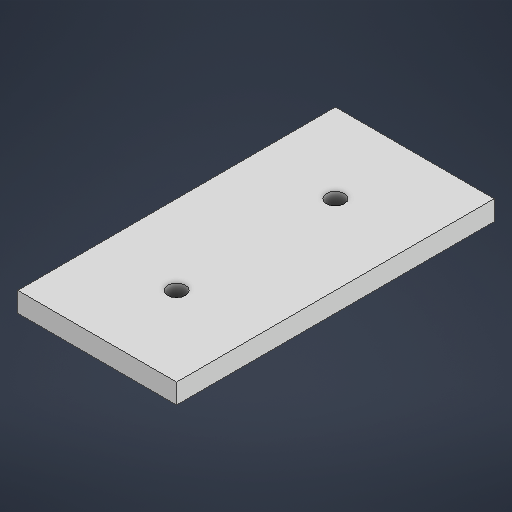
# Autodesk Inventor part: Bolt Slot Covers
Saved by Autodesk Inventor 2026.2 (Build 302298000, 298)
## iProperties
Created: 2026-05-27
Part Number: Bolt Slot Covers
Material: Generic
Document SubType Name: Modeling
Designer: mayhe
Density: 1 g/cm^3
Appearance: Default
Author: mayhe
Autodesk Inventor part; units mm, degrees
ref_plane "YZ Plane" through (0, 0, 0) normal (1, 0, 0) x (0, 1, 0)
ref_plane "XZ Plane" through (0, 0, 0) normal (0, 1, 0) x (-1, 0, 0)
ref_plane "XY Plane" through (0, 0, 0) normal (0, 0, 1) x (1, 0, 0)
sketch "Sketch1" plane through (0, 0, 0) normal (0, 1, 0) x (-1, 0, 0)
  line L0 (20, 40) -> (-20, 40)
  line L1 (-20, 40) -> (-20, -40)
  line L2 (-20, -40) -> (20, -40)
  line L3 (20, -40) -> (20, 40)
  line L4 (20, 40) -> (-20, -40) construction
  line L5 (-20, 40) -> (20, -40) construction
  circle A0 centre (0, 20) radius 2.25
  line L6 (20, 0) -> (36.628, 0)
  circle A1 centre (0, -20) radius 2.25
  point P0 (0, 0)
  dimension "d0" = 40
  dimension "d1" = 80
  dimension "d2" = 4.5
  dimension "d3" = 20
  constraints: 14 end point, 3 midpoint, 2 centre point, 2 horizontal, 2 parallel, 1 perpendicular, 1 symmetric about line, 1 other
  measures "d0" distance of L2.end L1.end
  measures "d1" distance of L1.end L0.end
  measures "d2" diameter of A0
  measures "d3" distance of point (0, 0) A0.centre
extrude "Extrusion1" add sketch "Sketch1" along normal mid plane 5
body "Solid1"
